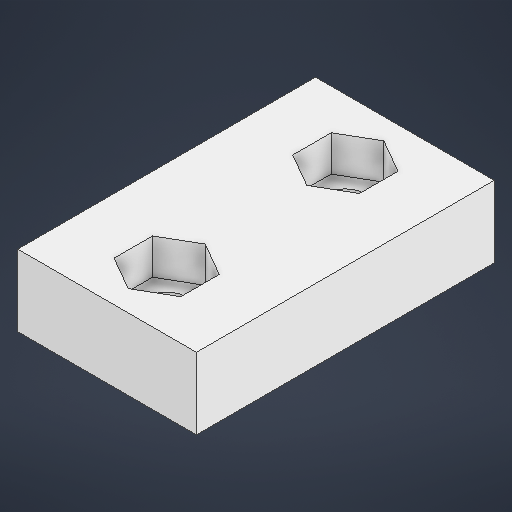
# Autodesk Inventor part: Dribbler Motor Mount Upper Section
Saved by Autodesk Inventor 2026.1 (Build 301233000, 233)
## iProperties
Created: 2025-12-08
Part Number: Dribbler Motor Mount Upper Section
Material: Generisch
Document SubType Name: Modeling
Designer: Familie
Density: 1 g/cm^3
Appearance: Weiß
Author: Familie
Autodesk Inventor part; units mm, degrees
ref_plane "YZ Plane" through (0, 0, 0) normal (1, 0, 0) x (0, 1, 0)
ref_plane "XZ Plane" through (0, 0, 0) normal (0, 1, 0) x (-1, 0, 0)
ref_plane "XY Plane" through (0, 0, 0) normal (0, 0, 1) x (1, 0, 0)
sketch "Skizze1" plane through (0, 0, 0) normal (0, 0, 1) x (1, 0, 0)
  line L0 (0, 0) -> (15, 0)
  line L1 (15, 0) -> (15, -25)
  line L2 (15, -25) -> (0, -25)
  line L3 (0, -25) -> (0, 0)
  line L4 (15.813, -10.2189) -> (15.812, -10.2179)
  line L5 (15.8113, -10.2187) -> (15.812, -10.2194)
  line L6 (15.812, -10.2179) -> (15.8113, -10.2187)
  line L7 (15.812, -10.2179) -> (15.8113, -10.2187)
  line L8 (15.812, -10.2179) -> (15.8113, -10.2187)
  line L9 (15.8113, -10.2187) -> (15.812, -10.2194)
  line L10 (15.8113, -10.2187) -> (15.812, -10.2194)
  line L11 (15.813, -10.2189) -> (15.812, -10.2179)
  line L12 (15.813, -10.2189) -> (15.812, -10.2179)
  line L13 (15.812, -10.2179) -> (15.8113, -10.2187)
  line L14 (15.813, -10.2189) -> (15.812, -10.2179)
  line L15 (15.8113, -10.2187) -> (15.812, -10.2194)
  line L16 (7.5, -8.2332) -> (4.7, -6.6166)
  line L17 (4.7, -6.6166) -> (4.7, -3.3834)
  line L18 (4.7, -3.3834) -> (7.5, -1.7668)
  line L19 (7.5, -1.7668) -> (10.3, -3.3834)
  line L20 (10.3, -3.3834) -> (10.3, -6.6166)
  line L21 (10.3, -6.6166) -> (7.5, -8.2332)
  circle A0 centre (7.5, -5) radius 1.6
  line L22 (10.3, -18.3834) -> (10.3, -21.6166)
  line L23 (10.3, -21.6166) -> (7.5, -23.2332)
  line L24 (7.5, -23.2332) -> (4.7, -21.6166)
  circle A1 centre (7.5, -20) radius 1.6
  line L25 (7.5, -16.7668) -> (10.3, -18.3834)
  line L26 (4.7, -18.3834) -> (7.5, -16.7668)
  line L27 (4.7, -21.6166) -> (4.7, -18.3834)
  dimension "d0" = 25
  dimension "d1" = 15
  dimension "d2" = 5.6
  dimension "d5" = 3.2
  dimension "d6" = 5.6
  dimension "d7" = 3.2
  dimension "d8" = 5
  dimension "d9" = 5
  dimension "d10" = 7.5
  constraints: 54 end point, 4 parallel, 2 centre point, 2 coincident, 1 horizontal, 1 perpendicular, 1 vertical alignment, 29 other
  measures "d0" distance of L0.end L1.end
  measures "d1" distance of L1.end L2.end
  measures "d2" distance between parallel lines of L17 L20
  measures "d5" diameter of A0
  measures "d6" distance between parallel lines of L26 L23
  measures "d7" diameter of A1
  measures "d8" distance from line of L0 A0.centre
  measures "d9" distance from line of L2 A1.centre
  measures "d10" distance from line of L1 A0.centre
extrude "Extrusion1" add sketch "Skizze1" along normal blind 6 contours L0 L1 L2 L3
extrude "Extrusion2" add sketch "Skizze1" along normal blind 3 contours L0 L1 L2 L3 | L16 L17 L18 L19 L20 L21 | L22 L23 L24 L27 L26 L25
equation "\"d9\" = d8"
